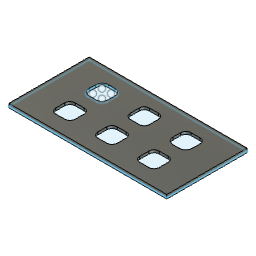
крыфшка v1 (Autodesk Fusion 360 design; units mm, degrees)
Autodesk Fusion 360 part; units mm, degrees
sketch "Sketch1" plane through (0, 0, 0) normal (0, 0, 1) x (1, 0, 0)
  line L0 (1, -1) -> (-121, -1)
  line L1 (-121, -1) -> (-121, 61)
  line L2 (-121, 61) -> (1, 61)
  line L3 (1, 61) -> (1, -1)
  constraint horizontal L0
  constraint vertical L1
  constraint horizontal L2
  constraint vertical L3
extrude "Extrude1" add sketch "Sketch1" along normal blind 5 makes body 1
shell "Shell1" thickness 1 removed faces 1 at (-39.6667, 19.6667, 5) on bodies 1
sketch "Sketch2" plane through (0, 0, 0) normal (0, 0, 1) x (1, 0, 0)
sketch "Sketch3" plane through (0, 0, 1) normal (0, 0, 1) x (-1, 0, 0)
  line L0 (0, -60) -> (120, -60)
  line L1 (120, -60) -> (120, 0)
  line L2 (120, 0) -> (0, 0)
  line L3 (0, 0) -> (0, -60)
  line L4 (89.0446, -34.9212) -> (96.0446, -34.9212)
  line L5 (100.0446, -38.9212) -> (100.0446, -45.9212)
  line L6 (96.0446, -49.9212) -> (89.0446, -49.9212)
  line L7 (85.0446, -45.9212) -> (85.0446, -38.9212)
  arc A0 (100.0446, -38.9212) -> (96.0446, -34.9212) centre (96.0446, -38.9212) ccw
  arc A1 (96.0446, -49.9212) -> (100.0446, -45.9212) centre (96.0446, -45.9212) ccw
  arc A2 (85.0446, -45.9212) -> (89.0446, -49.9212) centre (89.0446, -45.9212) ccw
  arc A3 (89.0446, -34.9212) -> (85.0446, -38.9212) centre (89.0446, -38.9212) ccw
  dimension "d4" = 4
  constraint tangent L4 A0
  constraint tangent L5 A0
  constraint tangent L5 A1
  constraint tangent L6 A1
  constraint equal A0 A1
  constraint tangent L6 A2
  constraint tangent L7 A2
  constraint equal A0 A2
  constraint tangent L4 A3
  constraint tangent L7 A3
  constraint equal A0 A3
  measures "d4" radius of A0
sketch "Sketch4" plane through (0, 0, 0) normal (0, 0, 1) x (1, 0, 0)
  line L0 (-63.5506, 50.1641) -> (-56.5506, 50.1641)
  line L1 (-52.5506, 46.1641) -> (-52.5506, 39.1641)
  line L2 (-56.5506, 35.1641) -> (-63.5506, 35.1641)
  line L3 (-67.5506, 39.1641) -> (-67.5506, 46.1641)
  arc A0 (-63.5506, 50.1641) -> (-67.5506, 46.1641) centre (-63.5506, 46.1641) ccw
  arc A1 (-52.5506, 46.1641) -> (-56.5506, 50.1641) centre (-56.5506, 46.1641) ccw
  arc A2 (-56.5506, 35.1641) -> (-52.5506, 39.1641) centre (-56.5506, 39.1641) ccw
  arc A3 (-67.5506, 39.1641) -> (-63.5506, 35.1641) centre (-63.5506, 39.1641) ccw
  dimension "d5" = 4
  constraint horizontal L0
  constraint vertical L1
  constraint horizontal L2
  constraint vertical L3
  constraint tangent L0 A0
  constraint tangent L3 A0
  constraint tangent L0 A1
  constraint tangent L1 A1
  constraint equal A0 A1
  constraint tangent L1 A2
  constraint tangent L2 A2
  constraint equal A0 A2
  constraint tangent L2 A3
  constraint tangent L3 A3
  constraint equal A0 A3
  measures "d5" radius of A0
sketch "Sketch5" plane through (0, 0, 0) normal (0, 0, 1) x (1, 0, 0)
  line L0 (-31.0562, 49.7368) -> (-24.0562, 49.7368)
  line L1 (-20.0562, 45.7368) -> (-20.0562, 39.7368)
  line L2 (-25.0562, 34.7368) -> (-30.0562, 34.7368)
  line L3 (-35.0562, 39.7368) -> (-35.0562, 45.7368)
  arc A0 (-31.0562, 49.7368) -> (-35.0562, 45.7368) centre (-31.0562, 45.7368) ccw
  arc A1 (-20.0562, 45.7368) -> (-24.0562, 49.7368) centre (-24.0562, 45.7368) ccw
  arc A2 (-35.0562, 39.7368) -> (-30.0562, 34.7368) centre (-30.0562, 39.7368) ccw
  arc A3 (-25.0562, 34.7368) -> (-20.0562, 39.7368) centre (-25.0562, 39.7368) ccw
  dimension "d6" = 4
  dimension "d7" = 5
  constraint horizontal L0
  constraint vertical L1
  constraint horizontal L2
  constraint vertical L3
  constraint tangent L0 A0
  constraint tangent L3 A0
  constraint tangent L0 A1
  constraint tangent L1 A1
  constraint equal A0 A1
  constraint tangent L2 A2
  constraint tangent L3 A2
  constraint tangent L1 A3
  constraint tangent L2 A3
  constraint equal A2 A3
  measures "d6" radius of A0
  measures "d7" radius of A2
sketch "Sketch6" plane through (0, 0, 0) normal (0, 0, 1) x (1, 0, 0)
  line L0 (-95.8036, 24.9793) -> (-88.8036, 24.9793)
  line L1 (-84.8036, 20.9793) -> (-84.8036, 13.9793)
  line L2 (-88.8036, 9.9793) -> (-95.8036, 9.9793)
  line L3 (-99.8036, 13.9793) -> (-99.8036, 20.9793)
  arc A0 (-95.8036, 24.9793) -> (-99.8036, 20.9793) centre (-95.8036, 20.9793) ccw
  arc A1 (-84.8036, 20.9793) -> (-88.8036, 24.9793) centre (-88.8036, 20.9793) ccw
  arc A2 (-88.8036, 9.9793) -> (-84.8036, 13.9793) centre (-88.8036, 13.9793) ccw
  arc A3 (-99.8036, 13.9793) -> (-95.8036, 9.9793) centre (-95.8036, 13.9793) ccw
  dimension "d8" = 4
  constraint horizontal L0
  constraint vertical L1
  constraint horizontal L2
  constraint vertical L3
  constraint tangent L0 A0
  constraint tangent L3 A0
  constraint tangent L0 A1
  constraint tangent L1 A1
  constraint equal A0 A1
  constraint tangent L1 A2
  constraint tangent L2 A2
  constraint equal A0 A2
  constraint tangent L2 A3
  constraint tangent L3 A3
  constraint equal A0 A3
  measures "d8" radius of A0
sketch "Sketch7" plane through (0, 0, 0) normal (0, 0, 1) x (1, 0, 0)
  line L0 (-63.4938, 25.1442) -> (-56.4938, 25.1442)
  line L1 (-52.4938, 21.1442) -> (-52.4938, 14.1442)
  line L2 (-56.4938, 10.1442) -> (-63.4938, 10.1442)
  line L3 (-67.4938, 14.1442) -> (-67.4938, 21.1442)
  arc A0 (-63.4938, 25.1442) -> (-67.4938, 21.1442) centre (-63.4938, 21.1442) ccw
  arc A1 (-52.4938, 21.1442) -> (-56.4938, 25.1442) centre (-56.4938, 21.1442) ccw
  arc A2 (-56.4938, 10.1442) -> (-52.4938, 14.1442) centre (-56.4938, 14.1442) ccw
  arc A3 (-67.4938, 14.1442) -> (-63.4938, 10.1442) centre (-63.4938, 14.1442) ccw
  dimension "d9" = 4
  constraint horizontal L0
  constraint vertical L1
  constraint horizontal L2
  constraint vertical L3
  constraint tangent L0 A0
  constraint tangent L3 A0
  constraint tangent L0 A1
  constraint tangent L1 A1
  constraint equal A0 A1
  constraint tangent L1 A2
  constraint tangent L2 A2
  constraint equal A0 A2
  constraint tangent L2 A3
  constraint tangent L3 A3
  constraint equal A0 A3
  measures "d9" radius of A0
sketch "Sketch8" plane through (0, 0, 0) normal (0, 0, 1) x (1, 0, 0)
  line L0 (-31.0303, 25.1442) -> (-24.0303, 25.1442)
  line L1 (-20.0303, 21.1442) -> (-20.0303, 14.1442)
  line L2 (-24.0303, 10.1442) -> (-31.0303, 10.1442)
  line L3 (-35.0303, 14.1442) -> (-35.0303, 21.1442)
  arc A0 (-31.0303, 25.1442) -> (-35.0303, 21.1442) centre (-31.0303, 21.1442) ccw
  arc A1 (-20.0303, 21.1442) -> (-24.0303, 25.1442) centre (-24.0303, 21.1442) ccw
  arc A2 (-24.0303, 10.1442) -> (-20.0303, 14.1442) centre (-24.0303, 14.1442) ccw
  arc A3 (-35.0303, 14.1442) -> (-31.0303, 10.1442) centre (-31.0303, 14.1442) ccw
  dimension "d10" = 4
  constraint horizontal L0
  constraint vertical L1
  constraint horizontal L2
  constraint vertical L3
  constraint tangent L0 A0
  constraint tangent L3 A0
  constraint tangent L0 A1
  constraint tangent L1 A1
  constraint equal A0 A1
  constraint tangent L1 A2
  constraint tangent L2 A2
  constraint equal A0 A2
  constraint tangent L2 A3
  constraint tangent L3 A3
  constraint equal A0 A3
  measures "d10" radius of A0
extrude "Extrude2" add sketch "Sketch1" along normal blind 2 separate body makes body 2
extrude "Extrude3" cut sketch "Sketch8" along normal blind 5 bodies 2
extrude "Extrude4" cut sketch "Sketch6" sketch "Sketch5" sketch "Sketch4" sketch "Sketch7" along normal blind 5 of sketch 2 of sketch 3 of sketch 4 bodies 2
sketch "Sketch9" plane through (0, 0, 0) normal (0, 0, 1) x (1, 0, 0)
  line L0 (-94.9607, 34.9419) -> (-89.9607, 34.9419)
  line L1 (-84.9607, 39.9419) -> (-84.9607, 44.9419)
  line L2 (-89.9607, 49.9419) -> (-94.9607, 49.9419)
  line L3 (-99.9607, 44.9419) -> (-99.9607, 39.9419)
  arc A0 (-99.9607, 39.9419) -> (-94.9607, 34.9419) centre (-94.9607, 39.9419) ccw
  arc A1 (-89.9607, 34.9419) -> (-84.9607, 39.9419) centre (-89.9607, 39.9419) ccw
  arc A2 (-84.9607, 44.9419) -> (-89.9607, 49.9419) centre (-89.9607, 44.9419) ccw
  arc A3 (-94.9607, 49.9419) -> (-99.9607, 44.9419) centre (-94.9607, 44.9419) ccw
  dimension "d17" = 5
  constraint horizontal L0
  constraint vertical L1
  constraint horizontal L2
  constraint vertical L3
  constraint tangent L0 A0
  constraint tangent L3 A0
  constraint tangent L0 A1
  constraint tangent L1 A1
  constraint equal A0 A1
  constraint tangent L1 A2
  constraint tangent L2 A2
  constraint equal A0 A2
  constraint tangent L2 A3
  constraint tangent L3 A3
  constraint equal A0 A3
  measures "d17" radius of A0
extrude "Extrude5" cut sketch "Sketch9" along normal blind 5 bodies 2
extrude "Extrude6" add sketch "Sketch1" against normal blind 1 thin wall 1 inside bodies 2
hidden bodies 1
